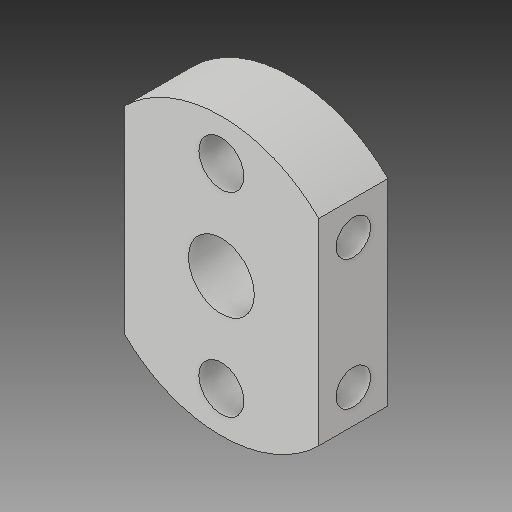
# Autodesk Inventor part: Part12
Saved by Autodesk Inventor 2019 (Build 230136000, 136)
## iProperties
Created: 2018-09-18
Part Number: Part12
Material: Generic
Document SubType Name: Modeling
Designer: drawing
Density: 1 g/cm^3
Appearance: Default
Author: drawing
Autodesk Inventor part; units mm, degrees
ref_plane "YZ Plane" through (0, 0, 0) normal (1, 0, 0) x (0, 1, 0)
ref_plane "XZ Plane" through (0, 0, 0) normal (0, 1, 0) x (-1, 0, 0)
sketch "Sketch1" plane through (0, 0, 0) normal (0, 0, 1) x (1, 0, 0)
  circle A0 centre (0, 0) radius 20.32
  dimension "d0" = 40.64
  constraints: 1 centre point, 1 coincident
  measures "d0" diameter of A0
extrude "Extrusion1" add sketch "Sketch1" along normal blind 10.16
sketch "Sketch2" plane through (0, 0, 10.16) normal (0, 0, 1) x (1, 0, 0)
  point P0 (0, 0)
  point P1 (0, 0)
  constraints: 1 coincident
hole "Hole1" at (0, 0, 10.16) direction (0, 0, -1) diameter 9.652 depth 10.9728 tip angle 118
sketch "Sketch3" plane through (0, 0, 10.16) normal (0, 0, 1) x (1, 0, 0)
  point P0 (0, 0)
  point P1 (0, 14.2875)
  point P2 (0, -14.2875)
  dimension "d10" = 28.575
  dimension "d11" = 14.2875
  constraints: 2 vertical alignment
  measures "d10" distance of point (0, 14.287) point (0, -14.287)
  measures "d11" distance of point (0, 0) point (0, 14.287)
hole "Hole2" at (0, 14.2875, 10.16) at (0, -14.2875, 10.16) direction (0, 0, -1) diameter 6.604 depth 10.9728 tip angle 118
sketch "Sketch4" plane through (0, 0, 10.16) normal (0, 0, 1) x (1, 0, 0)
  line L0 (-14.2875, -38.2443) -> (14.2875, -38.2443)
  line L1 (14.2875, -38.2443) -> (14.2875, 37.8114)
  line L2 (14.2875, 37.8114) -> (-14.2875, 37.8114)
  line L3 (-14.2875, 37.8114) -> (-14.2875, -38.2443)
  line L4 (-54.4025, 52.7865) -> (43.8573, 52.7865)
  line L5 (43.8573, 52.7865) -> (43.8573, -66.4941)
  line L6 (43.8573, -66.4941) -> (-54.4025, -66.4941)
  line L7 (-54.4025, -66.4941) -> (-54.4025, 52.7865)
  point P0 (0, 0)
  dimension "d19" = 28.575
  dimension "d20" = 14.2875
  constraints: 16 end point, 4 parallel, 2 horizontal, 2 perpendicular
  measures "d19" distance of L1.end L2.end
  measures "d20" distance from line of L3 point (0, 0)
extrude "Extrusion2" cut sketch "Sketch4" against normal blind 10.16
sketch "Sketch5" plane through (-14.2875, -14.4489, 10.16) normal (-1, 0, 0) x (0, 0, 1)
  line L0 (0, 0) -> (-10.16, 0) projected
  line L1 (0, 28.8977) -> (0, 0) projected
  line L2 (-10.16, 28.8977) -> (0, 28.8977) projected
  line L3 (-10.16, 0) -> (-10.16, 28.8977) projected
  point P0 (-10.16, 14.4489)
  point P1 (-5.08, 23.9739)
  point P2 (-5.08, 4.9239)
  dimension "d23" = 10.16
  dimension "d24" = 5.08
  dimension "d25" = 5.08
  dimension "d26" = 19.05
  dimension "d27" = 28.8977
  dimension "d28" = 4.9239
  measures "d23" distance of L2.start L1.start
  measures "d24" distance from line of L1 point (-5.08, 23.974)
  measures "d25" distance from line of L1 point (-5.08, 4.924)
  measures "d26" distance of point (-5.08, 4.924) point (-5.08, 23.974)
  measures "d27" distance of L0.end L2.start
  measures "d28" distance from line of L2 point (-5.08, 23.974)
hole "Hole3" at (-14.2875, 9.525, 5.08) at (-14.2875, -9.525, 5.08) direction (1, 0, 0) diameter 5.08 depth 10.9728 tip angle 118
ref_plane "Work Plane1" through (0, -14.4489, 10.16) normal (1, 0, 0) x (0, 0, -1)
mirror "Mirror1" about plane through (0, -14.4489, 10.16) normal (1, 0, 0) of "Hole3"
equation "\"d11\" = 0.5 * d10"
equation "\"d20\" = 0.5 * d19"
equation "\"d24\" = 0.5 * d23"
equation "\"d25\" = d24"
equation "\"d28\" = -0.5 * d26 + 0.5 * d27"
body "Solid1"
